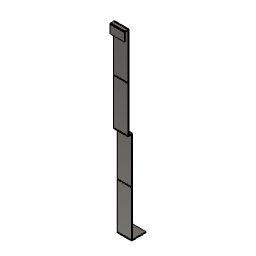
phone_stand2 (Autodesk Fusion 360 design; units mm, degrees)
Autodesk Fusion 360 part; units mm, degrees
sketch "Sketch1" plane through (0, 0, 0) normal (0, 0, 1) x (1, 0, 0)
  line L0 (80, 20) -> (80, 0)
  line L1 (-80, 30) -> (-80, 10)
  line L2 (-70, 30) -> (-70, 20)
  line L3 (-70, 0) -> (-70, 10)
  line L4 (-60, 30) -> (-60, 20)
  line L5 (-60, 0) -> (-60, 10)
  line L6 (-50, 30) -> (-50, 20)
  line L7 (-50, 0) -> (-50, 10)
  line L8 (-40, 30) -> (-40, 20)
  line L9 (-40, 0) -> (-40, 10)
  line L10 (-30, 30) -> (-30, 20)
  line L11 (-30, 0) -> (-30, 10)
  line L12 (-20, 30) -> (-20, 20)
  line L13 (-20, 0) -> (-20, 10)
  line L14 (-10, 30) -> (-10, 20)
  line L15 (-10, 0) -> (-10, 10)
  line L16 (0, 30) -> (0, 20)
  line L17 (0, 0) -> (0, 10)
  line L18 (10, 30) -> (10, 20)
  line L19 (10, 0) -> (10, 10)
  line L20 (20, 30) -> (20, 20)
  line L21 (20, 0) -> (20, 10)
  line L22 (30, 30) -> (30, 20)
  line L23 (30, 0) -> (30, 10)
  line L24 (40, 30) -> (40, 20)
  line L25 (40, 0) -> (40, 10)
  line L26 (50, 30) -> (50, 20)
  line L27 (50, 0) -> (50, 10)
  line L28 (60, 30) -> (60, 20)
  line L29 (60, 0) -> (60, 10)
  line L30 (70, 30) -> (70, 20)
  line L31 (70, 0) -> (70, 10)
  line L32 (-60, 20) -> (-70, 20)
  line L33 (-40, 20) -> (-50, 20)
  line L34 (-20, 20) -> (-30, 20)
  line L35 (0, 20) -> (-10, 20)
  line L36 (20, 20) -> (10, 20)
  line L37 (40, 20) -> (30, 20)
  line L38 (60, 20) -> (50, 20)
  line L39 (80, 20) -> (70, 20)
  line L40 (-70, 10) -> (-80, 10)
  line L41 (-50, 10) -> (-60, 10)
  line L42 (-30, 10) -> (-40, 10)
  line L43 (-10, 10) -> (-20, 10)
  line L44 (10, 10) -> (0, 10)
  line L45 (30, 10) -> (20, 10)
  line L46 (50, 10) -> (40, 10)
  line L47 (70, 10) -> (60, 10)
  line L48 (-70, 0) -> (-60, 0)
  line L49 (-50, 0) -> (-40, 0)
  line L50 (-30, 0) -> (-20, 0)
  line L51 (-10, 0) -> (0, 0)
  line L52 (10, 0) -> (20, 0)
  line L53 (30, 0) -> (40, 0)
  line L54 (50, 0) -> (60, 0)
  line L55 (70, 0) -> (80, 0)
  line L56 (60, 30) -> (70, 30)
  line L57 (0, 30) -> (10, 30)
  line L58 (40, 30) -> (50, 30)
  line L59 (20, 30) -> (30, 30)
  line L60 (-10, 30) -> (-20, 30)
  line L61 (-30, 30) -> (-40, 30)
  line L62 (-50, 30) -> (-60, 30)
  line L63 (-70, 30) -> (-80, 30)
  constraint horizontal L60
  constraint parallel L57 L60
sketch "Sketch5" plane through (0, 0, 0) normal (0, 0, 1) x (1, 0, 0)
  line L0 (80, -190) -> (-80, -190)
  line L1 (-80, -190) -> (-80, -90)
  line L2 (-70, -100) -> (-70, -90)
  line L3 (-60, -100) -> (-60, -90)
  line L4 (-60, -100) -> (-70, -100)
  line L5 (-50, -100) -> (-50, -90)
  line L6 (-40, -100) -> (-40, -90)
  line L7 (-40, -100) -> (-50, -100)
  line L8 (-30, -100) -> (-30, -90)
  line L9 (-20, -100) -> (-20, -90)
  line L10 (-20, -100) -> (-30, -100)
  line L11 (-10, -100) -> (-10, -90)
  line L12 (0, -100) -> (0, -90)
  line L13 (0, -100) -> (-10, -100)
  line L14 (10, -100) -> (10, -90)
  line L15 (20, -100) -> (20, -90)
  line L16 (20, -100) -> (10, -100)
  line L17 (30, -100) -> (30, -90)
  line L18 (40, -100) -> (40, -90)
  line L19 (40, -100) -> (30, -100)
  line L20 (50, -100) -> (50, -90)
  line L21 (60, -100) -> (60, -90)
  line L22 (60, -100) -> (50, -100)
  line L23 (70, -100) -> (70, -90)
  line L24 (80, -100) -> (70, -100)
  line L25 (-70, -90) -> (-80, -90)
  line L26 (-50, -90) -> (-60, -90)
  line L27 (-30, -90) -> (-40, -90)
  line L28 (-10, -90) -> (-20, -90)
  line L29 (10, -90) -> (0, -90)
  line L30 (30, -90) -> (20, -90)
  line L31 (50, -90) -> (40, -90)
  line L32 (70, -90) -> (60, -90)
  line L33 (80, -100) -> (80, -190)
  dimension "d17" = 100
  constraint horizontal L0
  constraint vertical L1
  constraint vertical L33
  measures "d17" distance of L1.end L0.end
sketch "Sketch8" plane through (0, 0, 0) normal (0, 0, 1) x (1, 0, 0)
  line L0 (80, 50) -> (70, 50)
  line L1 (70, 50) -> (70, 60)
  line L2 (60, 60) -> (70, 60)
  line L3 (60, 50) -> (60, 60)
  line L4 (60, 50) -> (50, 50)
  line L5 (50, 50) -> (50, 60)
  line L6 (40, 60) -> (50, 60)
  line L7 (40, 50) -> (40, 60)
  line L8 (40, 50) -> (30, 50)
  line L9 (30, 50) -> (30, 60)
  line L10 (20, 60) -> (30, 60)
  line L11 (20, 50) -> (20, 60)
  line L12 (20, 50) -> (10, 50)
  line L13 (10, 50) -> (10, 60)
  line L14 (0, 60) -> (10, 60)
  line L15 (0, 50) -> (0, 60)
  line L16 (0, 50) -> (-10, 50)
  line L17 (-10, 50) -> (-10, 60)
  line L18 (-20, 60) -> (-10, 60)
  line L19 (-20, 50) -> (-20, 60)
  line L20 (-20, 50) -> (-30, 50)
  line L21 (-30, 50) -> (-30, 60)
  line L22 (-40, 60) -> (-30, 60)
  line L23 (-40, 50) -> (-40, 60)
  line L24 (-40, 50) -> (-50, 50)
  line L25 (-50, 50) -> (-50, 60)
  line L26 (-60, 60) -> (-50, 60)
  line L27 (-60, 50) -> (-60, 60)
  line L28 (-60, 50) -> (-70, 50)
  line L29 (-70, 50) -> (-70, 60)
  line L30 (-80, 60) -> (-70, 60)
  line L31 (80, 50) -> (80, 560)
  line L32 (-80, 60) -> (-80, 570)
  line L33 (70, 560) -> (80, 560)
  line L34 (70, 560) -> (70, 570)
  line L35 (60, 560) -> (60, 570)
  line L36 (70, 570) -> (60, 570)
  line L37 (50, 560) -> (60, 560)
  line L38 (50, 560) -> (50, 570)
  line L39 (40, 560) -> (40, 570)
  line L40 (50, 570) -> (40, 570)
  line L41 (30, 560) -> (40, 560)
  line L42 (30, 560) -> (30, 570)
  line L43 (20, 560) -> (20, 570)
  line L44 (30, 570) -> (20, 570)
  line L45 (10, 560) -> (20, 560)
  line L46 (10, 560) -> (10, 570)
  line L47 (0, 560) -> (0, 570)
  line L48 (10, 570) -> (0, 570)
  line L49 (-10, 560) -> (0, 560)
  line L50 (-10, 560) -> (-10, 570)
  line L51 (-20, 560) -> (-20, 570)
  line L52 (-10, 570) -> (-20, 570)
  line L53 (-30, 560) -> (-20, 560)
  line L54 (-30, 560) -> (-30, 570)
  line L55 (-40, 560) -> (-40, 570)
  line L56 (-30, 570) -> (-40, 570)
  line L57 (-50, 560) -> (-40, 560)
  line L58 (-50, 560) -> (-50, 570)
  line L59 (-60, 560) -> (-60, 570)
  line L60 (-50, 570) -> (-60, 570)
  line L61 (-70, 560) -> (-60, 560)
  line L62 (-70, 560) -> (-70, 570)
  line L63 (-80, 560) -> (-80, 570)
  line L64 (-70, 570) -> (-80, 570)
  line L65 (70, 1110) -> (80, 1110)
  line L66 (50, 1110) -> (60, 1110)
  line L67 (30, 600) -> (30, 610)
  line L68 (50, 1120) -> (40, 1120)
  line L69 (80, 600) -> (70, 600)
  line L70 (20, 600) -> (10, 600)
  line L71 (20, 1110) -> (20, 1120)
  line L72 (50, 1110) -> (50, 1120)
  line L73 (10, 1120) -> (0, 1120)
  line L74 (0, 610) -> (10, 610)
  line L75 (30, 1120) -> (20, 1120)
  line L76 (60, 600) -> (50, 600)
  line L77 (-50, 1110) -> (-40, 1110)
  line L78 (40, 600) -> (30, 600)
  line L79 (-20, 1110) -> (-20, 1120)
  line L80 (10, 600) -> (10, 610)
  line L81 (-40, 1110) -> (-40, 1120)
  line L82 (-40, 600) -> (-50, 600)
  line L83 (-30, 1110) -> (-30, 1120)
  line L84 (0, 1110) -> (0, 1120)
  line L85 (-10, 1120) -> (-20, 1120)
  line L86 (70, 1110) -> (70, 1120)
  line L87 (-10, 1110) -> (-10, 1120)
  line L88 (-30, 1120) -> (-40, 1120)
  line L89 (-10, 1110) -> (0, 1110)
  line L90 (-70, 1110) -> (-60, 1110)
  line L91 (-30, 1110) -> (-20, 1110)
  line L92 (-60, 1110) -> (-60, 1120)
  line L93 (-50, 1120) -> (-60, 1120)
  line L94 (-50, 1110) -> (-50, 1120)
  line L95 (40, 1110) -> (40, 1120)
  line L96 (-70, 1120) -> (-80, 1120)
  line L97 (-40, 610) -> (-30, 610)
  line L98 (-20, 600) -> (-30, 600)
  line L99 (-20, 610) -> (-10, 610)
  line L100 (-70, 1110) -> (-70, 1120)
  line L101 (-70, 600) -> (-70, 610)
  line L102 (-30, 600) -> (-30, 610)
  line L103 (10, 1110) -> (10, 1120)
  line L104 (70, 1120) -> (60, 1120)
  line L105 (0, 600) -> (-10, 600)
  line L106 (-20, 600) -> (-20, 610)
  line L107 (-80, 610) -> (-80, 1120)
  line L108 (40, 600) -> (40, 610)
  line L109 (80, 600) -> (80, 1110)
  line L110 (-40, 600) -> (-40, 610)
  line L111 (-60, 600) -> (-70, 600)
  line L112 (70, 600) -> (70, 610)
  line L113 (50, 600) -> (50, 610)
  line L114 (-50, 600) -> (-50, 610)
  line L115 (40, 610) -> (50, 610)
  line L116 (30, 1110) -> (40, 1110)
  line L117 (0, 600) -> (0, 610)
  line L118 (-60, 610) -> (-50, 610)
  line L119 (60, 610) -> (70, 610)
  line L120 (-10, 600) -> (-10, 610)
  line L121 (-80, 610) -> (-70, 610)
  line L122 (60, 1110) -> (60, 1120)
  line L123 (-60, 600) -> (-60, 610)
  line L124 (60, 600) -> (60, 610)
  line L125 (10, 1110) -> (20, 1110)
  line L126 (20, 600) -> (20, 610)
  line L127 (20, 610) -> (30, 610)
  line L128 (30, 1110) -> (30, 1120)
  constraint perpendicular L0 L31
  constraint perpendicular L30 L32
  constraint perpendicular L69 L109
  constraint perpendicular L107 L121
sketch "Sketch9" plane through (0, 0, 0) normal (0, 0, 1) x (1, 0, 0)
  line L0 (-80, 1145) -> (-80, 1295)
  line L1 (80, 1135) -> (80, 1295)
  line L2 (80, 1295) -> (-80, 1295)
  line L3 (80, 1135) -> (80, 1145)
  line L4 (70, 1135) -> (80, 1135)
  line L5 (70, 1135) -> (70, 1145)
  line L6 (60, 1135) -> (70, 1135)
  line L7 (60, 1135) -> (60, 1145)
  line L8 (60, 1145) -> (70, 1145)
  line L9 (50, 1135) -> (60, 1135)
  line L10 (50, 1135) -> (50, 1145)
  line L11 (40, 1135) -> (40, 1145)
  line L12 (40, 1145) -> (50, 1145)
  line L13 (30, 1135) -> (40, 1135)
  line L14 (30, 1135) -> (30, 1145)
  line L15 (20, 1135) -> (20, 1145)
  line L16 (20, 1145) -> (30, 1145)
  line L17 (10, 1135) -> (20, 1135)
  line L18 (10, 1135) -> (10, 1145)
  line L19 (0, 1135) -> (0, 1145)
  line L20 (0, 1145) -> (10, 1145)
  line L21 (-10, 1135) -> (0, 1135)
  line L22 (-10, 1135) -> (-10, 1145)
  line L23 (-20, 1135) -> (-20, 1145)
  line L24 (-20, 1145) -> (-10, 1145)
  line L25 (-30, 1135) -> (-20, 1135)
  line L26 (-30, 1135) -> (-30, 1145)
  line L27 (-40, 1135) -> (-40, 1145)
  line L28 (-40, 1145) -> (-30, 1145)
  line L29 (-50, 1135) -> (-40, 1135)
  line L30 (-50, 1135) -> (-50, 1145)
  line L31 (-60, 1135) -> (-60, 1145)
  line L32 (-60, 1145) -> (-50, 1145)
  line L33 (-70, 1135) -> (-60, 1135)
  line L34 (-70, 1135) -> (-70, 1145)
  line L35 (-80, 1145) -> (-70, 1145)
  constraint coincident L1 L3.end
sketch "Sketch10" plane through (0, 0, 0) normal (0, 0, 1) x (1, 0, 0)
  line L0 (-80, -70) -> (-80, -30)
  line L1 (80, -40) -> (80, -80)
  line L2 (70, -70) -> (70, -80)
  line L3 (70, -80) -> (80, -80)
  line L4 (70, -40) -> (70, -30)
  line L5 (70, -40) -> (80, -40)
  line L6 (60, -70) -> (70, -70)
  line L7 (60, -70) -> (60, -80)
  line L8 (60, -30) -> (70, -30)
  line L9 (60, -40) -> (60, -30)
  line L10 (50, -70) -> (50, -80)
  line L11 (50, -80) -> (60, -80)
  line L12 (50, -40) -> (50, -30)
  line L13 (50, -40) -> (60, -40)
  line L14 (40, -70) -> (50, -70)
  line L15 (40, -70) -> (40, -80)
  line L16 (40, -30) -> (50, -30)
  line L17 (40, -40) -> (40, -30)
  line L18 (30, -70) -> (30, -80)
  line L19 (30, -80) -> (40, -80)
  line L20 (30, -40) -> (30, -30)
  line L21 (30, -40) -> (40, -40)
  line L22 (20, -70) -> (30, -70)
  line L23 (20, -70) -> (20, -80)
  line L24 (20, -30) -> (30, -30)
  line L25 (20, -40) -> (20, -30)
  line L26 (10, -70) -> (10, -80)
  line L27 (10, -80) -> (20, -80)
  line L28 (10, -40) -> (10, -30)
  line L29 (10, -40) -> (20, -40)
  line L30 (0, -70) -> (10, -70)
  line L31 (0, -70) -> (0, -80)
  line L32 (0, -30) -> (10, -30)
  line L33 (0, -40) -> (0, -30)
  line L34 (-10, -70) -> (-10, -80)
  line L35 (-10, -80) -> (0, -80)
  line L36 (-10, -40) -> (-10, -30)
  line L37 (-10, -40) -> (0, -40)
  line L38 (-20, -70) -> (-10, -70)
  line L39 (-20, -70) -> (-20, -80)
  line L40 (-20, -30) -> (-10, -30)
  line L41 (-20, -40) -> (-20, -30)
  line L42 (-30, -70) -> (-30, -80)
  line L43 (-30, -80) -> (-20, -80)
  line L44 (-30, -40) -> (-30, -30)
  line L45 (-30, -40) -> (-20, -40)
  line L46 (-40, -70) -> (-30, -70)
  line L47 (-40, -70) -> (-40, -80)
  line L48 (-40, -30) -> (-30, -30)
  line L49 (-40, -40) -> (-40, -30)
  line L50 (-50, -70) -> (-50, -80)
  line L51 (-50, -80) -> (-40, -80)
  line L52 (-50, -40) -> (-50, -30)
  line L53 (-50, -40) -> (-40, -40)
  line L54 (-60, -70) -> (-50, -70)
  line L55 (-60, -70) -> (-60, -80)
  line L56 (-60, -30) -> (-50, -30)
  line L57 (-60, -40) -> (-60, -30)
  line L58 (-70, -70) -> (-70, -80)
  line L59 (-70, -80) -> (-60, -80)
  line L60 (-70, -40) -> (-70, -30)
  line L61 (-70, -40) -> (-60, -40)
  line L62 (-80, -70) -> (-70, -70)
  line L63 (-80, -30) -> (-70, -30)
  line L64 (-80, -40) -> (-80, -30)
extrude "Extrude1" add sketch "Sketch5" along normal blind 10 makes body 1
extrude "Extrude2" add sketch "Sketch10" along normal blind 10 separate body makes body 2
extrude "Extrude3" add sketch "Sketch8" along normal blind 10 separate body contours L0 L1 L2 L3 L4 L5 L6 L7 L8 L9 L10 L11 L12 L13 L14 L15 L16 L17 L18 L19 L20 L21 L22 L23 L24 L25 L26 L27 L28 L29 L30 L31 L32 L33 L34 L35 L36 L37 L38 L39 L40 L41 L42 L43 L44 L45 L46 L47 L48 L49 L50 L51 L52 L53 L54 L55 L56 L57 L58 L59 L60 L61 L62 L63 L64 makes body 3
extrude "Extrude4" add sketch "Sketch8" along normal blind 10 separate body contours L65 L66 L67 L68 L69 L70 L71 L72 L73 L74 L75 L76 L77 L78 L79 L80 L81 L82 L83 L84 L85 L86 L87 L88 L89 L90 L91 L92 L93 L94 L95 L96 L97 L98 L99 L100 L101 L102 L103 L104 L105 L106 L107 L108 L109 L110 L111 L112 L113 L114 L115 L116 L117 L118 L119 L120 L121 L122 L123 L124 L125 L126 L127 L128 makes body 4
extrude "Extrude5" add sketch "Sketch9" along normal blind 10 separate body contours L0 L1 L2 L3 L4 L5 L7 L8 L9 L10 L11 L12 L13 L14 L15 L16 L17 L18 L19 L20 L21 L22 L23 L24 L25 L26 L27 L28 L29 L30 L31 L32 L33 L34 L35 makes body 5
copy_body "CopyPasteBodies1" bodies 3 makes body 6
move_body "Move1" bodies 6 to x (1, 0, 0) y (0, 1, 0) z (0, 0, 1) at (-200, 0, 0)
copy_body "CopyPasteBodies2" bodies 4 makes body 7
move_body "Move2" bodies 7 to x (1, 0, 0) y (0, 1, 0) z (0, 0, 1) at (-200, 0, 0)
copy_body "CopyPasteBodies3" bodies 2 makes body 8
move_body "Move3" bodies 8 to x (1, 0, 0) y (0, 1, 0) z (0, 0, 1) at (-200, 0, 0)
move_body "Move4" bodies 1 to x (1, 0, 0) y (0, 0, 1) z (0, -1, 0) at (0, -70, 100)
move_body "Move5" bodies 3 to x (1, 0, 0) y (0, 0, -1) z (0, 1, 0) at (0, -40, 60)
move_body "Move6" bodies 8 to x (1, 0, 0) y (0, 1, 0) z (0, 0, 1) at (200, -245, -510)
move_body "Move7" bodies 8 to x (1, 0, 0) y (0, 1, 0) z (0, 0, 1) at (0, 285, 0)
move_body "Move8" bodies 6 to x (1, 0, 0) y (0, 0, -1) z (0, 1, 0) at (200, 0, -450)
move_body "Move9" bodies 8 2 6 3 1 to x (1, 0, 0) y (0, 1, 0) z (0, 0, 1) at (0, 0, 500)
move_body "Move10" bodies 8 6 7 to x (1, 0, 0) y (0, 1, 0) z (0, 0, 1) at (0, 400, 0)
move_body "Move11" bodies 4 to x (1, 0, 0) y (0, 0, -1) z (0, 1, 0) at (0, -40, 600)
move_body "Move12" bodies 6 8 to x (1, 0, 0) y (0, 1, 0) z (0, 0, 1) at (0, -400, -510)
move_body "Move13" bodies 7 to x (1, 0, 0) y (0, 0, -1) z (0, 1, 0) at (200, 0, -20)
move_body "Move14" bodies 5 to x (1, 0, 0) y (0, 1, 0) z (0, 0, 1) at (0, -1135, -1540)
move_body "Move15" bodies 8 2 4 3 5 1 6 7 to x (1, 0, 0) y (0, 1, 0) z (0, 0, 1) at (0, 0, 500)
